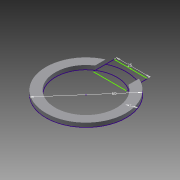
# Autodesk Inventor part: ServoHornLayer
Saved by Autodesk Inventor 2016 (Build 200138000, 138)
## iProperties
Created: 2015-05-10
Part Number: ServoHornLayer
Material: Generic
Document SubType Name: Modeling
Designer: Erin
Density: 1 g/cm^3
Appearance: Default
Author: Erin
Autodesk Inventor part; units mm, degrees
ref_plane "YZ Plane" through (0, 0, 0) normal (1, 0, 0) x (0, 1, 0)
ref_plane "XZ Plane" through (0, 0, 0) normal (0, 1, 0) x (-1, 0, 0)
ref_plane "XY Plane" through (0, 0, 0) normal (0, 0, 1) x (1, 0, 0)
sketch "Sketch1" plane through (0, 0, 0) normal (0, 0, 1) x (1, 0, 0)
  circle A0 centre (0, 0) radius 30
  circle A1 centre (0, 0) radius 23
  line L0 (-12.5, 33.563) -> (12.5, 33.563)
  line L1 (12.5, 33.563) -> (12.5, 17.72)
  line L2 (12.5, 17.72) -> (-12.5, 17.72)
  line L3 (-12.5, 17.72) -> (-12.5, 33.563)
  point P0 (0, 33.563)
  dimension "d0" = 60
  dimension "d1" = 7
  dimension "d4" = 25
  constraints: 8 end point, 2 centre point, 2 coincident, 2 parallel, 1 horizontal, 1 midpoint, 1 perpendicular, 1 vertical alignment
  measures "d0" diameter of A0
  measures "d1" radial gap between concentric circles of A1 A0
  measures "d4" distance of L0.start L0.end
extrude "Extrusion1" add sketch "Sketch1" along normal blind 3 contours A0 L3 A1 L1 | L1 A1 L3 A0
extrude "Extrusion2" cut sketch "Sketch1" along normal blind 3 contours L1 A1 L3 A0 | A0 L3 L0 L1 | L1 L2 L3 A1 picked at (8.89, 26.0762) picked at (0.8791, 19.4294)
body "Solid1"
